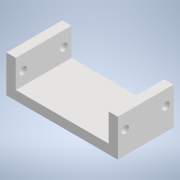
# Autodesk Inventor part: Part1
Saved by Autodesk Inventor 2022 (Build 260153070, 153G)
## iProperties
Created: 2021-07-07
Part Number: Part1
Material: Generic
Document SubType Name: Modeling
Designer: Bhagiratha
Density: 1 g/cm^3
Appearance: Default
Author: Bhagiratha
Autodesk Inventor part; units mm, degrees
ref_plane "YZ Plane" through (0, 0, 0) normal (1, 0, 0) x (0, 1, 0)
ref_plane "XZ Plane" through (0, 0, 0) normal (0, 1, 0) x (-1, 0, 0)
ref_plane "XY Plane" through (0, 0, 0) normal (0, 0, 1) x (1, 0, 0)
sketch "Sketch2" plane through (0, 0, 0) normal (0, 1, 0) x (-1, 0, 0)
  line L0 (-76.2, -38.1) -> (76.2, -38.1)
  line L1 (76.2, -38.1) -> (76.2, 38.1)
  line L2 (76.2, 38.1) -> (-76.2, 38.1)
  line L3 (-76.2, 38.1) -> (-76.2, -38.1)
  line L4 (-76.2, -38.1) -> (76.2, 38.1) construction
  line L5 (76.2, -38.1) -> (-76.2, 38.1) construction
  point P0 (0, 0)
  dimension "d0" = 152.4
  dimension "d1" = 76.2
  constraints: 12 end point, 2 midpoint, 2 parallel, 1 horizontal, 1 perpendicular
  measures "d0" distance of L2.end L1.end
  measures "d1" distance of L1.end L0.end
extrude "Extrusion1" add sketch "Sketch2" along normal blind 50.8
sketch "Sketch3" plane through (0, 50.8, 0) normal (0, 1, 0) x (1, 0, 0)
  line L0 (63.5, -38.1) -> (-63.5, -38.1)
  line L1 (-63.5, -38.1) -> (-63.5, 38.1)
  line L2 (-63.5, 38.1) -> (63.5, 38.1)
  line L3 (63.5, 38.1) -> (63.5, -38.1)
  line L4 (63.5, -38.1) -> (-63.5, 38.1) construction
  line L5 (-63.5, -38.1) -> (63.5, 38.1) construction
  point P0 (0, 0)
  dimension "d4" = 127
  dimension "d5" = 76.2
  constraints: 12 end point, 2 midpoint, 2 parallel, 1 horizontal, 1 perpendicular
  measures "d4" distance of L1.end L2.end
  measures "d5" distance of L0.end L1.end
extrude "Extrusion2" cut sketch "Sketch3" against normal blind 38.1
sketch "Sketch4" plane through (63.5, 50.8, -38.1) normal (-1, 0, 0) x (0, 0, 1)
  line L0 (0, 0) -> (76.2, 0) projected
  line L1 (0, -38.1) -> (0, 0) projected
  point P0 (38.1, -50.8)
  point P1 (10.16, -20.32)
  dimension "d8" = 20.32
  dimension "d9" = 10.16
  measures "d8" distance from line of L0 point (10.16, -20.32)
  measures "d9" distance from line of L1 point (10.16, -20.32)
hole "Hole1" at (63.5, 30.48, -27.94) direction (1, 0, 0) diameter 10 end through all
sketch "Sketch5" plane through (63.5, 50.8, -38.1) normal (-1, 0, 0) x (0, 0, 1)
  line L0 (0, 0) -> (76.2, 0) projected
  line L1 (76.2, 0) -> (76.2, -38.1) projected
  point P0 (38.1, -50.8)
  point P1 (66.04, -20.32)
  dimension "d17" = 20.32
  dimension "d18" = 10.16
  measures "d17" distance from line of L0 point (66.04, -20.32)
  measures "d18" distance from line of L1 point (66.04, -20.32)
hole "Hole2" at (63.5, 30.48, 27.94) direction (1, 0, 0) diameter 10 end through all
sketch "Sketch6" plane through (-63.5, 50.8, 38.1) normal (1, 0, 0) x (0, 0, -1)
  line L0 (0, 0) -> (76.2, 0) projected
  line L1 (0, -38.1) -> (0, 0) projected
  line L2 (76.2, 0) -> (76.2, -38.1) projected
  point P0 (38.1, -50.8)
  point P1 (10.16, -20.32)
  point P2 (66.04, -20.32)
  dimension "d26" = 20.32
  dimension "d27" = 10.16
  dimension "d28" = 20.32
  dimension "d29" = 10.16
  measures "d26" distance from line of L0 point (10.16, -20.32)
  measures "d27" distance from line of L1 point (10.16, -20.32)
  measures "d28" distance from line of L0 point (66.04, -20.32)
  measures "d29" distance from line of L2 point (66.04, -20.32)
hole "Hole3" at (-63.5, 30.48, 27.94) at (-63.5, 30.48, -27.94) direction (-1, 0, 0) diameter 10 end through all
sketch "Sketch7" plane through (63.5, 50.8, -38.1) normal (-1, 0, 0) x (0, 0, 1)
  line L0 (0, 0) -> (76.2, 0) projected
  line L1 (0, -38.1) -> (0, 0) projected
  point P0 (38.1, -50.8)
  point P1 (37, -20.32)
  dimension "d37" = 20.32
  dimension "d38" = 37
  measures "d37" distance from line of L0 point (37, -20.32)
  measures "d38" distance from line of L1 point (37, -20.32)
hole "Hole4" at (63.5, 30.48, -1.1) direction (1, 0, 0) diameter 10 end through all
sketch "Sketch8" plane through (-76.2, 0, -38.1) normal (-1, 0, 0) x (0, 0, 1)
  line L0 (0, 50.8) -> (76.2, 50.8) projected
  line L1 (0, 0) -> (0, 50.8) projected
  point P0 (38.1, 0)
  point P1 (37, 30.48)
  dimension "d46" = 20.32
  dimension "d47" = 37
  measures "d46" distance from line of L0 point (37, 30.48)
  measures "d47" distance from line of L1 point (37, 30.48)
hole "Hole5" at (-76.2, 30.48, -1.1) direction (1, 0, 0) diameter 10 end through all
body "Solid1"
